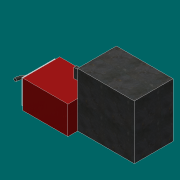
# Autodesk Inventor part: Welder
Saved by Autodesk Inventor 2017 (Build 210142000, 142)
## iProperties
Created: 2018-01-23
Part Number: Welder
Material: Steel
Document SubType Name: Modeling
Designer: Graeme_Van_Dongen
Density: 7.85 g/cm^3
Appearance: Plate
Author: Graeme_Van_Dongen
Autodesk Inventor part; units mm, degrees
ref_plane "YZ Plane" through (0, 0, 0) normal (1, 0, 0) x (0, 1, 0)
sketch "Sketch1" plane through (0, 0, 0) normal (1, 0, 0) x (0, 1, 0)
  line L0 (0, 120.65) -> (184.15, 120.65)
  line L1 (184.15, 120.65) -> (184.15, -120.65)
  line L2 (184.15, -120.65) -> (0, -120.65)
  line L3 (0, -120.65) -> (0, 120.65)
  point P0 (0, 0)
  point P1 (0, 0)
  dimension "d0" = 184.15
  dimension "d1" = 241.3
  constraints: 8 end point, 2 parallel, 1 coincident, 1 horizontal, 1 midpoint, 1 perpendicular
  measures "d0" distance of L1.end L2.end
  measures "d1" distance of L0.end L1.end
extrude "Extrusion1" add sketch "Sketch1" along normal blind 295.275
sketch "Sketch2" plane through (0, 0, 0) normal (-1, 0, 0) x (0, 0, 1)
  line L0 (120.65, 0) -> (120.65, 184.15) construction
  line L1 (120.65, 184.15) -> (-120.65, 184.15) construction
  line L2 (-120.65, 184.15) -> (-120.65, 0) construction
  line L3 (-120.65, 0) -> (120.65, 0) construction
  line L4 (-107.95, 171.45) -> (107.95, 171.45)
  line L5 (107.95, 171.45) -> (107.95, 12.7)
  line L6 (107.95, 12.7) -> (-107.95, 12.7)
  line L7 (-107.95, 12.7) -> (-107.95, 171.45)
  point P0 (0, 0)
  dimension "d4" = 12.7
  constraints: 8 end point, 3 other
  measures "d4" distance between parallel lines of L1 L4
extrude "Extrusion2" add sketch "Sketch2" along normal blind 19.05
ref_plane "Work Plane1" through (0, 104.775, 0) normal (0, 1, 0) x (-1, 0, 0)
sketch "Sketch3" plane through (0, 104.775, 0) normal (0, 1, 0) x (-1, 0, 0)
  line L0 (0, 120.65) -> (0, -120.65) construction
  line L1 (133.2378, 0) -> (-22.2063, 0) construction
  line L2 (0, 0) -> (19.05, 0)
  arc A0 (19.05, 0) -> (95.25, 76.2) centre (19.05, 76.2) ccw
  dimension "d8" = 19.05
  dimension "d22" = 76.2
  constraints: 2 end point, 2 point on circle, 1 centre point, 1 horizontal alignment, 1 point on line, 1 tangent
  measures "d8" distance of L2.start L2.end
  measures "d22" radius of A0
sketch "Sketch4" plane through (0, 0, 0) normal (-1, 0, 0) x (0, 0, 1)
  circle A0 centre (0, 104.775) radius 9.525
  point P0 (0, 0)
  dimension "d9" = 19.05
  constraints: 1 centre point, 1 coincident
  measures "d9" diameter of A0
sweep "Sweep1" add profiles "Sketch4" path "Sketch3"
sketch "Sketch5" plane through (0, 0, 0) normal (0, 1, 0) x (-1, 0, 0)
  line L0 (-295.275, 120.65) -> (-295.275, -120.65) construction
  line L1 (-295.275, 57.15) -> (-666.75, 57.15)
  line L2 (-666.75, 57.15) -> (-666.75, -196.85)
  line L3 (-666.75, -196.85) -> (-295.275, -196.85)
  line L4 (-295.275, -196.85) -> (-295.275, 57.15)
  line L5 (0, -120.65) -> (0, 120.65) construction
  point P0 (0, 0)
  dimension "d12" = 666.75
  dimension "d13" = 76.2
  dimension "d14" = 254
  constraints: 8 end point, 2 parallel, 1 horizontal, 1 perpendicular, 1 point on line
  measures "d12" distance between parallel lines of L2 L5
  measures "d13" distance from line of L0.end L3
  measures "d14" distance of L1.end L2.end
extrude "Extrusion3" add sketch "Sketch5" along normal blind 355.6
sketch "Sketch6" plane through (0, 0, 0) normal (0, 1, 0) x (-1, 0, 0)
  line L0 (-168.275, -63.5) -> (-295.275, -63.5)
  line L1 (-295.275, -63.5) -> (-295.275, -44.45)
  line L2 (-295.275, -44.45) -> (-168.275, -44.45)
  line L3 (-168.275, -44.45) -> (-168.275, -63.5)
  line L4 (-295.275, -196.85) -> (-295.275, 57.15) construction
  line L5 (0, -120.65) -> (-295.275, -120.65) construction
  point P0 (0, 0)
  dimension "d17" = 127
  dimension "d18" = 19.05
  dimension "d19" = 57.15
  constraints: 8 end point, 2 parallel, 1 collinear, 1 horizontal, 1 perpendicular
  measures "d17" distance of L1.end L2.end
  measures "d18" distance of L0.end L1.end
  measures "d19" distance between parallel lines of L5 L0
extrude "Extrusion4" add sketch "Sketch6" along normal blind 247.65
ref_plane "Work Plane2" through (295.275, 0, -196.85) normal (-1, 0, 0) x (0, 0, 1)
split_face "Split1"
body "Solid1"
